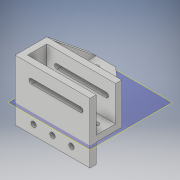
# Autodesk Inventor part: xIdler
Saved by Autodesk Inventor 2019 (Build 230136000, 136)
## iProperties
Created: 2019-05-16
Part Number: xIdler
Material: Generic
Document SubType Name: Modeling
Designer: Alex Jones
Density: 1 g/cm^3
Appearance: Default
Author: Alex Jones
Autodesk Inventor part; units mm, degrees
ref_plane "YZ Plane" through (0, 0, 0) normal (1, 0, 0) x (0, 1, 0)
ref_plane "XZ Plane" through (0, 0, 0) normal (0, 1, 0) x (-1, 0, 0)
ref_plane "XY Plane" through (0, 0, 0) normal (0, 0, 1) x (1, 0, 0)
sketch "Sketch1" plane through (0, 0, 0) normal (0, 1, 0) x (-1, 0, 0)
  line L0 (-25.4, -25.4) -> (25.4, -25.4) construction
  line L1 (25.4, -25.4) -> (25.4, 25.4) construction
  line L2 (25.4, 25.4) -> (-25.4, 25.4) construction
  line L3 (-25.4, 25.4) -> (-25.4, -25.4) construction
  line L4 (-25.4, -25.4) -> (25.4, 25.4) construction
  line L5 (25.4, -25.4) -> (-25.4, 25.4) construction
  line L6 (-25.4, 25.4) -> (25.4, 25.4) construction
  line L7 (25.4, 25.4) -> (25.4, 45.4) construction
  line L8 (25.4, 45.4) -> (-25.4, 45.4)
  line L9 (-25.4, 45.4) -> (-25.4, 25.4) construction
  line L10 (25.4, 45.4) -> (45.4, 45.4)
  line L11 (45.4, 45.4) -> (45.4, -25.4)
  line L12 (45.4, -25.4) -> (25.4, -25.4) construction
  line L13 (25.4, -25.4) -> (25.4, 25.4) construction
  line L14 (25.4, 25.4) -> (25.4, 45.4) construction
  line L15 (-25.4, 45.4) -> (45.4, 45.4)
  line L16 (51.75, 45.4) -> (51.75, 51.75)
  line L17 (51.75, 51.75) -> (-25.4, 51.75)
  line L18 (-25.4, 51.75) -> (-25.4, 45.4)
  line L19 (51.75, 45.4) -> (45.4, 45.4) construction
  line L20 (45.4, 45.4) -> (45.4, -25.4)
  line L21 (45.4, -25.4) -> (51.75, -25.4)
  line L22 (51.75, -25.4) -> (51.75, 45.4)
  line L23 (45.4, 45.4) -> (51.75, 45.4) construction
  point P0 (0, 0)
  dimension "d0" = 50.8
  dimension "d1" = 20
  dimension "d2" = 20
  dimension "d3" = 6.35
  dimension "d4" = 6.35
  constraints: 48 end point, 12 parallel, 7 perpendicular, 6 horizontal, 2 midpoint
  measures "d0" distance of L0.end L1.end
  measures "d1" distance of L11.end L12.end
  measures "d2" distance of L8.end L2.end
  measures "d3" distance of L11.end L21.end
  measures "d4" distance of L17.end L8.end
extrude "Extrusion1" add sketch "Sketch1" along normal blind 62.3
sketch "Sketch2" plane through (-51.75, 0, 51.75) normal (0, 0, 1) x (1, 0, 0)
  line L0 (6.35, 0) -> (0, 0) projected
  line L1 (77.15, 0) -> (77.15, 62.3) projected
  line L2 (0, 0) -> (77.15, 0)
  line L3 (77.15, 0) -> (77.15, 20)
  line L4 (77.15, 20) -> (0, 20)
  line L5 (0, 20) -> (0, 0)
  line L6 (0, 0) -> (0, 62.3) projected
  line L7 (0, 10) -> (77.15, 10) construction
  circle A0 centre (19.05, 10) radius 2.75
  circle A1 centre (38.575, 10) radius 2.75
  circle A2 centre (58.1, 10) radius 2.75
  point P0 (51.75, 0)
  dimension "d7" = 20
  dimension "d8" = 5.5
  dimension "d9" = 19.05
  dimension "d12" = 19.525
  constraints: 10 end point, 3 centre point, 3 point on line, 2 horizontal, 2 parallel, 1 midpoint, 1 perpendicular, 4 other
  measures "d7" distance between parallel lines of L2 L4
  measures "d8" diameter of A0
  measures "d9" distance from line of L5 A0.centre
  measures "d12" distance of A0.centre A1.centre
extrude "Extrusion2" cut sketch "Sketch2" against normal blind 62.3 contours A0 | A1 | A2
sketch "Sketch3" plane through (-51.75, 0, -25.4) normal (-1, 0, 0) x (0, 0, 1)
  circle A0 centre (19.05, 10) radius 2.75
  line L0 (0, 0) -> (77.15, 0) projected
  line L1 (0, 0) -> (0, 62.3) projected
  circle A1 centre (38.575, 10) radius 2.75
  circle A2 centre (58.1, 10) radius 2.75
  point P0 (25.4, 0)
  dimension "d19" = 10
  dimension "d20" = 5.5
  dimension "d21" = 19.05
  dimension "d24" = 19.525
  constraints: 3 centre point, 1 horizontal, 4 other
  measures "d19" distance from line of L0 A0.centre
  measures "d20" diameter of A0
  measures "d21" distance from line of L1 A0.centre
  measures "d24" distance of A0.centre A1.centre
extrude "Extrusion3" cut sketch "Sketch3" against normal blind 62.3
ref_plane "Work Plane1" through (0, 20, 0) normal (0, -1, 0) x (1, 0, 0)
sketch "Sketch4" plane through (0, 20, 0) normal (0, -1, 0) x (1, 0, 0)
  line L0 (-45.4, -25.4) -> (-51.75, -25.4) projected
  line L1 (-45.4, 45.4) -> (-45.4, -25.4) projected
  line L2 (25.4, 45.4) -> (-45.4, 45.4) projected
  line L3 (25.4, 51.75) -> (25.4, 45.4) projected
  line L4 (-51.75, 51.75) -> (25.4, 51.75) projected
  line L5 (-51.75, -25.4) -> (-51.75, 51.75) projected
  line L6 (-45.4, 45.4) -> (-45.4, -25.4) projected
  line L7 (-45.4, 45.4) -> (-25.4, 45.4)
  line L8 (-25.4, 45.4) -> (-25.4, 25.4) construction
  line L9 (-25.4, -25.4) -> (-45.4, -25.4)
  line L10 (-45.4, -25.4) -> (-45.4, 45.4)
  line L11 (25.4, 45.4) -> (-45.4, 45.4) projected
  line L12 (25.4, 45.4) -> (-25.4, 45.4)
  line L13 (-25.4, 45.4) -> (-25.4, 25.4) construction
  line L14 (-25.4, 25.4) -> (25.4, 25.4) construction
  line L15 (25.4, 25.4) -> (25.4, 45.4)
  line L16 (-25.4, 25.4) -> (-25.4, -25.4) construction
  line L17 (25.4, 35.4) -> (-45.4, 35.4) construction
  line L18 (-35.4, -25.4) -> (-35.4, 45.4) construction
  circle A0 centre (-35.4, 35.4) radius 2.75
  circle A1 centre (-10, 35.4) radius 2.75
  circle A2 centre (15.4, 35.4) radius 2.75
  circle A3 centre (-35.4, 10) radius 2.75
  circle A4 centre (-35.4, -15.4) radius 2.75
  line L19 (25.4, 25.4) -> (25.4, 19.05)
  line L20 (25.4, 19.05) -> (-25.4, -25.4)
  point P0 (0, 0)
  dimension "d32" = 20
  dimension "d35" = 25.4
  dimension "d40" = 5.5
  dimension "d43" = 25.4
  dimension "d50" = 6.35
  constraints: 26 end point, 6 perpendicular, 5 centre point, 5 parallel, 4 point on line, 3 horizontal, 2 midpoint, 2 vertical, 8 other
  measures "d32" distance of L14.end L2.start
  measures "d35" distance of A0.centre A1.centre
  measures "d40" diameter of A0
  measures "d43" distance of A0.centre A3.centre
  measures "d50" distance of L14.end L19.end
extrude "Extrusion4" add sketch "Sketch4" against normal blind 6.35 contours L1 L2 L15 L19 L20 L9
sketch "Sketch5" plane through (0, 26.35, 0) normal (0, 1, 0) x (1, 0, 0)
  line L0 (25.4, -45.4) -> (25.4, -19.05) projected
  line L1 (-45.4, -45.4) -> (-45.4, 25.4) projected
  line L2 (25.4, -19.05) -> (-45.4, -19.05)
  line L3 (-45.4, -19.05) -> (-45.4, -25.4)
  line L4 (-45.4, -25.4) -> (25.4, -25.4)
  line L5 (25.4, -25.4) -> (25.4, -19.05)
  point P0 (0, 0)
  dimension "d51" = 6.35
  constraints: 8 end point, 2 parallel, 1 horizontal, 1 perpendicular, 1 point on line
  measures "d51" distance between parallel lines of L4 L2
extrude "Extrusion5" add sketch "Sketch5" along normal up to surface (35.95 mm away)
sketch "Sketch6" plane through (25.4, 26.35, 19.05) normal (0, 0, -1) x (-1, 0, 0)
  line L0 (-27.427, 21) -> (85.8592, 21) construction
  line L1 (0, 0) -> (50.8, 0) projected
  line L2 (7.113, 21) -> (62.913, 21) construction
  line L3 (9.613, 23.5) -> (60.413, 23.5)
  line L4 (60.413, 18.5) -> (9.613, 18.5)
  arc A0 (9.613, 23.5) -> (9.613, 18.5) centre (9.613, 21) ccw
  arc A1 (60.413, 18.5) -> (60.413, 23.5) centre (60.413, 21) ccw
  point P0 (25.4, -26.35)
  point P1 (35.013, 21)
  dimension "d54" = 21
  dimension "d55" = 5
  dimension "d56" = 50.8
  constraints: 10 end point, 6 point on circle, 4 point on line, 4 tangent, 2 centre point, 1 horizontal, 1 midpoint, 1 parallel
  measures "d54" distance between parallel lines of L1 L0
  measures "d55" distance between parallel lines of L4 L3
  measures "d56" distance of L3.start L3.end
extrude "Extrusion6" cut sketch "Sketch6" against normal through all
sketch "Sketch7" plane through (-45.4, 26.35, -25.4) normal (1, 0, 0) x (0, 0, -1)
  line L0 (-44.45, 35.95) -> (0, 35.95) projected
  line L1 (-44.45, 35.95) -> (0, 35.95)
  line L2 (0, 0) -> (0, 35.95) projected
  line L3 (0, 35.95) -> (0, 0)
  line L4 (0, 0) -> (-44.45, 35.95)
  point P0 (-25.4, -26.35)
  constraints: 6 end point, 1 collinear, 1 perpendicular
extrude "Extrusion7" cut sketch "Sketch7" against normal through all
body "Solid1"
